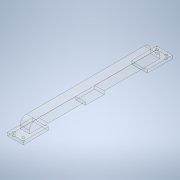
# Autodesk Inventor part: IndexRailM
Saved by Autodesk Inventor 2022 (Build 260153000, 153)
## iProperties
Created: 2022-01-13
Part Number: IndexRailM
Material: Polycarbonate, Clear
Document SubType Name: Modeling
Designer: tagaz
Density: 1.2 g/cm^3
Appearance: Polycarbonate - Clear
Author: tagaz
Autodesk Inventor part; units mm, degrees
ref_plane "YZ Plane" through (0, 0, 0) normal (1, 0, 0) x (0, 1, 0)
ref_plane "XZ Plane" through (0, 0, 0) normal (0, 1, 0) x (-1, 0, 0)
ref_plane "XY Plane" through (0, 0, 0) normal (0, 0, 1) x (1, 0, 0)
sketch "Sketch1" plane through (0, 0, 0) normal (1, 0, 0) x (0, 1, 0)
  line L0 (0, 0) -> (0, 0)
  line L1 (25.4, 0) -> (25.4, 12.7)
  line L2 (12.7, 25.4) -> (0, 25.4)
  line L3 (0, 25.4) -> (0, 0)
  line L4 (12.7, -238.6076) -> (0, -238.6076)
  line L5 (0, -238.6076) -> (0, -213.2076)
  line L6 (0, -213.2076) -> (0, -213.2076)
  line L7 (25.4, -213.2076) -> (25.4, -225.9076)
  arc A0 (25.4, 12.7) -> (12.7, 25.4) centre (12.7, 12.7) ccw
  arc A1 (12.7, -238.6076) -> (25.4, -225.9076) centre (12.7, -225.9076) ccw
  arc A2 (6.35, -12.7) -> (0, 0) centre (-8.8867, -12.3808) ccw
  arc A3 (0, -213.2076) -> (6.35, -200.5076) centre (-8.8867, -200.8268) ccw
  line L8 (25.4, 0) -> (25.4, -213.2076)
  line L9 (6.35, -200.5076) -> (6.35, -12.7)
  point P0 (0, -213.2076)
  point P1 (0, -213.2076)
  dimension "d5" = 25.4
  dimension "d6" = 12.7
  dimension "d9" = 264.0076
  dimension "d10" = 25.4
  dimension "d12" = 25.4
  dimension "d15" = 15.24
  dimension "d16" = 15.24
  constraints: 20 end point, 8 point on circle, 5 parallel, 4 centre point, 3 tangent, 2 horizontal, 2 perpendicular, 1 coincident, 1 vertical
  measures "d5" distance of L4.end L5.end
  measures "d6" radius of A0
  measures "d9" distance between parallel lines of L2 L4
  measures "d10" distance between parallel lines of L0 L2
  measures "d12" distance between parallel lines of L7 L5
  measures "d15" radius of A2
  measures "d16" radius of A3
extrude "Extrusion1" add sketch "Sketch1" along normal mid plane 19.05
sketch "Sketch2" plane through (-9.525, 0, 0) normal (0, -1, 0) x (1, 0, 0)
  line L0 (0, 0) -> (19.05, 0) projected
  line L1 (19.05, 12.7) -> (19.05, 25.4) projected
  line L2 (0, 0) -> (19.05, 0)
  line L3 (19.05, 0) -> (19.05, 25.4)
  line L4 (19.05, 25.4) -> (0, 25.4)
  line L5 (0, 25.4) -> (0, 0)
  line L6 (0, -213.2076) -> (19.05, -213.2076) projected
  line L7 (0, -238.6076) -> (19.05, -238.6076) projected
  line L8 (19.05, -213.2076) -> (0, -213.2076)
  line L9 (0, -213.2076) -> (0, -238.6076)
  line L10 (0, -238.6076) -> (19.05, -238.6076)
  line L11 (19.05, -238.6076) -> (19.05, -213.2076)
  line L12 (25.4, -206.8576) -> (-6.35, -206.8576)
  line L13 (-6.35, -206.8576) -> (-6.35, -244.9576)
  line L14 (25.4, -244.9576) -> (25.4, -206.8576)
  line L15 (-6.35, -6.35) -> (25.4, -6.35)
  line L16 (25.4, -6.35) -> (25.4, 31.75)
  line L17 (-6.35, 31.75) -> (-6.35, -6.35)
  line L18 (-6.35, 44.45) -> (25.4, 44.45)
  line L19 (25.4, 44.45) -> (25.4, 31.75)
  line L20 (-6.35, 31.75) -> (-6.35, 44.45)
  line L21 (-6.35, -244.9576) -> (-6.35, -257.6576)
  line L22 (-6.35, -257.6576) -> (25.4, -257.6576)
  line L23 (25.4, -257.6576) -> (25.4, -244.9576)
  point P0 (9.525, 0)
  dimension "d17" = 31.75
  dimension "d18" = 38.1
  dimension "d19" = 31.75
  dimension "d20" = 38.1
  dimension "d23" = 12.7
  constraints: 40 end point, 7 parallel, 7 perpendicular, 5 horizontal, 1 vertical
  measures "d17" distance of L14.start L13.end
  measures "d18" distance of L13.end L12.end
  measures "d19" distance of L17.start L16.end
  measures "d20" distance of L16.end L15.end
  measures "d23" distance of L13.end L21.end
extrude "Extrusion2" add sketch "Sketch2" against normal blind 6.35 contours L5 L4 L1 L3 L0 | L6 L11 L7 L9 | L14 L23 L22 L21 L13 L12 | L17 L20 L18 L19 L16 L15
sketch "Sketch3" plane through (-9.525, 6.35, 0) normal (0, 1, 0) x (1, 0, 0)
  circle A0 centre (0, 251.3076) radius 2.54
  circle A1 centre (19.05, 251.3076) radius 2.54
  line L0 (25.4, 206.8576) -> (25.4, 257.6576) projected
  line L1 (25.4, 257.6576) -> (-6.35, 257.6576) projected
  line L2 (-6.35, 257.6576) -> (-6.35, 206.8576) projected
  circle A2 centre (0, -38.1) radius 2.54
  circle A3 centre (19.05, -38.1) radius 2.54
  line L3 (-6.35, 6.35) -> (-6.35, -44.45) projected
  line L4 (-6.35, -44.45) -> (25.4, -44.45) projected
  line L5 (25.4, -44.45) -> (25.4, 6.35) projected
  point P0 (9.525, 0)
  dimension "d24" = 5.08
  dimension "d25" = 5.08
  dimension "d26" = 6.35
  dimension "d27" = 6.35
  dimension "d28" = 6.35
  dimension "d29" = 6.35
  dimension "d30" = 5.08
  dimension "d31" = 5.08
  dimension "d32" = 6.35
  dimension "d33" = 6.35
  dimension "d34" = 6.35
  dimension "d35" = 6.35
  constraints: 4 centre point
  measures "d24" diameter of A0
  measures "d25" diameter of A1
  measures "d26" distance from line of A1.centre L0
  measures "d27" distance from line of A1.centre L1
  measures "d28" distance from line of L1 A0.centre
  measures "d29" distance from line of A0.centre L2
  measures "d30" diameter of A2
  measures "d31" diameter of A3
  measures "d32" distance from line of A2.centre L3
  measures "d33" distance from line of L4 A2.centre
  measures "d34" distance from line of L4 A3.centre
  measures "d35" distance from line of L5 A3.centre
extrude "Extrusion3" cut sketch "Sketch3" against normal through all
sketch "Sketch4" plane through (9.525, 0, 0) normal (1, 0, 0) x (0, 0, -1)
  line L0 (200.5076, 6.35) -> (12.7, 6.35) projected
  line L1 (87.5538, 0) -> (125.6538, 0)
  line L2 (125.6538, 0) -> (125.6538, 6.35)
  line L3 (125.6538, 6.35) -> (87.5538, 6.35)
  line L4 (87.5538, 6.35) -> (87.5538, 0)
  line L5 (87.5538, 0) -> (125.6538, 6.35) construction
  line L6 (125.6538, 0) -> (87.5538, 6.35) construction
  point P0 (0, 0)
  point P1 (106.6038, 6.35)
  point P2 (106.6038, 3.175)
  dimension "d38" = 38.1
  constraints: 12 end point, 3 midpoint, 2 parallel, 1 horizontal, 1 perpendicular, 1 point on line
  measures "d38" distance of L3.end L2.end
extrude "Extrusion4" add sketch "Sketch4" against normal blind 19.05
body "Solid1"
